Autodesk Fusion 360 part; units mm, degrees
(part 9 of 9)
  line L288 (-3.2885, -31.7147) -> (2.6698, -31.7147) construction
  line L289 (2.6698, -31.7147) -> (2.6698, -21.1314) construction
  line L290 (2.6698, -21.1314) -> (-3.2885, -21.1314) construction
  line L291 (-3.2885, -21.1314) -> (-3.2885, -31.7147) construction
  line L292 (13.3802, -31.7147) -> (19.3488, -31.7147) construction
  line L293 (19.3488, -31.7147) -> (19.3488, -21.1314) construction
  line L294 (19.3488, -21.1314) -> (13.3802, -21.1314) construction
  line L295 (13.3802, -21.1314) -> (13.3802, -31.7147) construction
  line L296 (30.049, -31.7147) -> (36.3121, -31.7147) construction
  line L297 (36.3121, -31.7147) -> (36.3121, -21.1314) construction
  line L298 (36.3121, -21.1314) -> (30.049, -21.1314) construction
  line L299 (30.049, -21.1314) -> (30.049, -31.7147) construction
  line L300 (46.7177, -31.7147) -> (53.3943, -31.7147) construction
  line L301 (53.3943, -31.7147) -> (53.3943, -21.1314) construction
  line L302 (53.3943, -21.1314) -> (46.7177, -21.1314) construction
  line L303 (46.7177, -21.1314) -> (46.7177, -31.7147) construction
  line L304 (63.3865, -31.7147) -> (69.0399, -31.7147) construction
  line L305 (69.0399, -31.7147) -> (69.0399, -21.1314) construction
  line L306 (69.0399, -21.1314) -> (63.3865, -21.1314) construction
  line L307 (63.3865, -21.1314) -> (63.3865, -31.7147) construction
  line L308 (80.0552, -31.7147) -> (81.0577, -31.7147) construction
  line L309 (81.0577, -31.7147) -> (81.0577, -21.1314) construction
  line L310 (81.0577, -21.1314) -> (80.0552, -21.1314) construction
  line L311 (80.0552, -21.1314) -> (80.0552, -31.7147) construction
  line L312 (-86.6323, -50.2147) -> (-80.643, -50.2147) construction
  line L313 (-80.643, -50.2147) -> (-80.643, -39.6314) construction
  line L314 (-80.643, -39.6314) -> (-86.6323, -39.6314) construction
  line L315 (-86.6323, -39.6314) -> (-86.6323, -50.2147) construction
  line L316 (-69.9635, -50.2147) -> (-60.2225, -50.2147) construction
  line L317 (-60.2225, -50.2147) -> (-60.2225, -39.6314) construction
  line L318 (-60.2225, -39.6314) -> (-69.9635, -39.6314) construction
  line L319 (-69.9635, -39.6314) -> (-69.9635, -50.2147) construction
  line L320 (-53.2948, -50.2147) -> (-47.6414, -50.2147) construction
  line L321 (-47.6414, -50.2147) -> (-47.6414, -39.6314) construction
  line L322 (-47.6414, -39.6314) -> (-53.2948, -39.6314) construction
  line L323 (-53.2948, -39.6314) -> (-53.2948, -50.2147) construction
  line L324 (-36.626, -50.2147) -> (-35.6235, -50.2147) construction
  line L325 (-35.6235, -50.2147) -> (-35.6235, -39.6314) construction
  line L326 (-35.6235, -39.6314) -> (-36.626, -39.6314) construction
  line L327 (-36.626, -39.6314) -> (-36.626, -50.2147) construction
  line L328 (-19.9573, -50.2147) -> (-13.9887, -50.2147) construction
  line L329 (-13.9887, -50.2147) -> (-13.9887, -39.6314) construction
  line L330 (-13.9887, -39.6314) -> (-19.9573, -39.6314) construction
  line L331 (-19.9573, -39.6314) -> (-19.9573, -50.2147) construction
  line L332 (-3.2885, -50.2147) -> (2.7421, -50.2147) construction
  line L333 (2.7421, -50.2147) -> (2.7421, -39.6314) construction
  line L334 (2.7421, -39.6314) -> (-3.2885, -39.6314) construction
  line L335 (-3.2885, -39.6314) -> (-3.2885, -50.2147) construction
  line L336 (13.3802, -50.2147) -> (14.3827, -50.2147) construction
  line L337 (14.3827, -50.2147) -> (14.3827, -39.6314) construction
  line L338 (14.3827, -39.6314) -> (13.3802, -39.6314) construction
  line L339 (13.3802, -39.6314) -> (13.3802, -50.2147) construction
  line L340 (30.049, -50.2147) -> (35.7024, -50.2147) construction
  line L341 (35.7024, -50.2147) -> (35.7024, -39.6314) construction
  line L342 (35.7024, -39.6314) -> (30.049, -39.6314) construction
  line L343 (30.049, -39.6314) -> (30.049, -50.2147) construction
  line L344 (46.7177, -50.2147) -> (52.4383, -50.2147) construction
  line L345 (52.4383, -50.2147) -> (52.4383, -39.6314) construction
  line L346 (52.4383, -39.6314) -> (46.7177, -39.6314) construction
  line L347 (46.7177, -39.6314) -> (46.7177, -50.2147) construction
  line L348 (63.3865, -50.2147) -> (69.0399, -50.2147) construction
  line L349 (69.0399, -50.2147) -> (69.0399, -39.6314) construction
  line L350 (69.0399, -39.6314) -> (63.3865, -39.6314) construction
  line L351 (63.3865, -39.6314) -> (63.3865, -50.2147) construction
  line L352 (80.0552, -50.2147) -> (86.0238, -50.2147) construction
  line L353 (86.0238, -50.2147) -> (86.0238, -39.6314) construction
  line L354 (86.0238, -39.6314) -> (80.0552, -39.6314) construction
  line L355 (80.0552, -39.6314) -> (80.0552, -50.2147) construction
  line L356 (-86.6323, -68.7148) -> (-80.9789, -68.7148) construction
  line L357 (-80.9789, -68.7148) -> (-80.9789, -58.1314) construction
  line L358 (-80.9789, -58.1314) -> (-86.6323, -58.1314) construction
  line L359 (-86.6323, -58.1314) -> (-86.6323, -68.7148) construction
  line L360 (-69.9635, -68.7148) -> (-65.23, -68.7148) construction
  line L361 (-65.23, -68.7148) -> (-65.23, -58.1314) construction
  line L362 (-65.23, -58.1314) -> (-69.9635, -58.1314) construction
  line L363 (-69.9635, -58.1314) -> (-69.9635, -68.7148) construction
  line L364 (-53.2948, -68.7148) -> (-48.184, -68.7148) construction
  line L365 (-48.184, -68.7148) -> (-48.184, -58.1314) construction
  line L366 (-48.184, -58.1314) -> (-53.2948, -58.1314) construction
  line L367 (-53.2948, -58.1314) -> (-53.2948, -68.7148) construction
  line L368 (-36.626, -68.7148) -> (-29.6962, -68.7148) construction
  line L369 (-29.6962, -68.7148) -> (-29.6962, -58.1314) construction
  line L370 (-29.6962, -58.1314) -> (-36.626, -58.1314) construction
  line L371 (-36.626, -58.1314) -> (-36.626, -68.7148) construction
  line L372 (-19.9573, -68.7148) -> (-18.9548, -68.7148) construction
  line L373 (-18.9548, -68.7148) -> (-18.9548, -58.1314) construction
  line L374 (-18.9548, -58.1314) -> (-19.9573, -58.1314) construction
  line L375 (-19.9573, -58.1314) -> (-19.9573, -68.7148) construction
  line L376 (-3.2885, -68.7148) -> (2.3649, -68.7148) construction
  line L377 (2.3649, -68.7148) -> (2.3649, -58.1314) construction
  line L378 (2.3649, -58.1314) -> (-3.2885, -58.1314) construction
  line L379 (-3.2885, -58.1314) -> (-3.2885, -68.7148) construction
  line L380 (13.3802, -68.7148) -> (20.0568, -68.7148) construction
  line L381 (20.0568, -68.7148) -> (20.0568, -58.1314) construction
  line L382 (20.0568, -58.1314) -> (13.3802, -58.1314) construction
  line L383 (13.3802, -58.1314) -> (13.3802, -68.7148) construction
  line L384 (30.049, -68.7148) -> (37.139, -68.7148) construction
  line L385 (37.139, -68.7148) -> (37.139, -58.1314) construction
  line L386 (37.139, -58.1314) -> (30.049, -58.1314) construction
  line L387 (30.049, -58.1314) -> (30.049, -68.7148) construction
  line L388 (46.7177, -68.7148) -> (53.415, -68.7148) construction
  line L389 (53.415, -68.7148) -> (53.415, -58.1314) construction
  line L390 (53.415, -58.1314) -> (46.7177, -58.1314) construction
  line L391 (46.7177, -58.1314) -> (46.7177, -68.7148) construction
  line L392 (63.3865, -68.7148) -> (69.3292, -68.7148) construction
  line L393 (69.3292, -68.7148) -> (69.3292, -58.1314) construction
  line L394 (69.3292, -58.1314) -> (63.3865, -58.1314) construction
  line L395 (63.3865, -58.1314) -> (63.3865, -68.7148) construction
  line L396 (80.0552, -68.7148) -> (86.06, -68.7148) construction
  line L397 (86.06, -68.7148) -> (86.06, -58.1314) construction
  line L398 (86.06, -58.1314) -> (80.0552, -58.1314) construction
  line L399 (80.0552, -58.1314) -> (80.0552, -68.7148) construction
  line L400 (-86.6323, -87.2148) -> (-80.6017, -87.2148) construction
  line L401 (-80.6017, -87.2148) -> (-80.6017, -76.6314) construction
  line L402 (-80.6017, -76.6314) -> (-86.6323, -76.6314) construction
  line L403 (-86.6323, -76.6314) -> (-86.6323, -87.2148) construction
  line L404 (-69.9635, -87.2148) -> (-64.3101, -87.2148) construction
  line L405 (-64.3101, -87.2148) -> (-64.3101, -76.6314) construction
  line L406 (-64.3101, -76.6314) -> (-69.9635, -76.6314) construction
  line L407 (-69.9635, -76.6314) -> (-69.9635, -87.2148) construction
  line L408 (-53.2948, -87.2148) -> (-46.5975, -87.2148) construction
  line L409 (-46.5975, -87.2148) -> (-46.5975, -76.6314) construction
  line L410 (-46.5975, -76.6314) -> (-53.2948, -76.6314) construction
  line L411 (-53.2948, -76.6314) -> (-53.2948, -87.2148) construction
  line L412 (-36.626, -87.2148) -> (-30.6833, -87.2148) construction
  line L413 (-30.6833, -87.2148) -> (-30.6833, -76.6314) construction
  line L414 (-30.6833, -76.6314) -> (-36.626, -76.6314) construction
  line L415 (-36.626, -76.6314) -> (-36.626, -87.2148) construction
  line L416 (-19.9573, -87.2148) -> (-13.9267, -87.2148) construction
  line L417 (-13.9267, -87.2148) -> (-13.9267, -76.6314) construction
  line L418 (-13.9267, -76.6314) -> (-19.9573, -76.6314) construction
  line L419 (-19.9573, -76.6314) -> (-19.9573, -87.2148) construction
  line L420 (-3.2885, -87.2148) -> (-2.286, -87.2148) construction
  line L421 (-2.286, -87.2148) -> (-2.286, -76.6314) construction
  line L422 (-2.286, -76.6314) -> (-3.2885, -76.6314) construction
  line L423 (-3.2885, -76.6314) -> (-3.2885, -87.2148) construction
  line L424 (13.3802, -87.2148) -> (19.3385, -87.2148) construction
  line L425 (19.3385, -87.2148) -> (19.3385, -76.6314) construction
  line L426 (19.3385, -76.6314) -> (13.3802, -76.6314) construction
  line L427 (13.3802, -76.6314) -> (13.3802, -87.2148) construction
  line L428 (30.049, -87.2148) -> (35.9917, -87.2148) construction
  line L429 (35.9917, -87.2148) -> (35.9917, -76.6314) construction
  line L430 (35.9917, -76.6314) -> (30.049, -76.6314) construction
  line L431 (30.049, -76.6314) -> (30.049, -87.2148) construction
  line L432 (46.7177, -87.2148) -> (53.3943, -87.2148) construction
  line L433 (53.3943, -87.2148) -> (53.3943, -76.6314) construction
  line L434 (53.3943, -76.6314) -> (46.7177, -76.6314) construction
  line L435 (46.7177, -76.6314) -> (46.7177, -87.2148) construction
  line L436 (63.3865, -87.2148) -> (70.3318, -87.2148) construction
  line L437 (70.3318, -87.2148) -> (70.3318, -76.6314) construction
  line L438 (70.3318, -76.6314) -> (63.3865, -76.6314) construction
  line L439 (63.3865, -76.6314) -> (63.3865, -87.2148) construction
  line L440 (80.0552, -87.2148) -> (85.7086, -87.2148) construction
  line L441 (85.7086, -87.2148) -> (85.7086, -76.6314) construction
  line L442 (85.7086, -76.6314) -> (80.0552, -76.6314) construction
  line L443 (80.0552, -76.6314) -> (80.0552, -87.2148) construction
sketch "Sketch6" plane through (0, 0, 7) normal (0, 0, 1) x (-1, 0, 0)
  line L0 (57.9, 38.615) -> (42.9, 38.615)
  line L1 (42.9, 38.615) -> (42.9, 53.615)
  line L2 (42.9, 53.615) -> (57.9, 53.615)
  line L3 (57.9, 53.615) -> (57.9, 38.615)
  line L4 (-9.3, 20.17) -> (-24.3, 20.17)
  line L5 (-24.3, 20.17) -> (-24.3, 35.17)
  line L6 (-24.3, 35.17) -> (-9.3, 35.17)
  line L7 (-9.3, 35.17) -> (-9.3, 20.17)
  line L8 (-26.1, 20.17) -> (-41.1, 20.17)
  line L9 (-41.1, 20.17) -> (-41.1, 35.17)
  line L10 (-41.1, 35.17) -> (-26.1, 35.17)
  line L11 (-26.1, 35.17) -> (-26.1, 20.17)
  line L12 (-42.9, 20.17) -> (-57.9, 20.17)
  line L13 (-57.9, 20.17) -> (-57.9, 35.17)
  line L14 (-57.9, 35.17) -> (-42.9, 35.17)
  line L15 (-42.9, 35.17) -> (-42.9, 20.17)
  line L16 (-59.7, 1.725) -> (-74.7, 1.725)
  line L17 (-74.7, 1.725) -> (-74.7, 16.725)
  line L18 (-74.7, 16.725) -> (-59.7, 16.725)
  line L19 (-59.7, 16.725) -> (-59.7, 1.725)
  line L20 (7.5, 1.725) -> (-7.5, 1.725)
  line L21 (-7.5, 1.725) -> (-7.5, 16.725)
  line L22 (-7.5, 16.725) -> (7.5, 16.725)
  line L23 (7.5, 16.725) -> (7.5, 1.725)
  line L24 (-59.7, 20.17) -> (-74.7, 20.17)
  line L25 (-74.7, 20.17) -> (-74.7, 35.17)
  line L26 (-74.7, 35.17) -> (-59.7, 35.17)
  line L27 (-59.7, 35.17) -> (-59.7, 20.17)
  line L28 (57.9, 1.725) -> (42.9, 1.725)
  line L29 (42.9, 1.725) -> (42.9, 16.725)
  line L30 (42.9, 16.725) -> (57.9, 16.725)
  line L31 (57.9, 16.725) -> (57.9, 1.725)
  line L32 (41.1, 38.615) -> (26.1, 38.615)
  line L33 (26.1, 38.615) -> (26.1, 53.615)
  line L34 (26.1, 53.615) -> (41.1, 53.615)
  line L35 (41.1, 53.615) -> (41.1, 38.615)
  line L36 (41.1, 1.725) -> (26.1, 1.725)
  line L37 (26.1, 1.725) -> (26.1, 16.725)
  line L38 (26.1, 16.725) -> (41.1, 16.725)
  line L39 (41.1, 16.725) -> (41.1, 1.725)
  line L40 (-76.5, 1.725) -> (-91.5, 1.725)
  line L41 (-91.5, 1.725) -> (-91.5, 16.725)
  line L42 (-91.5, 16.725) -> (-76.5, 16.725)
  line L43 (-76.5, 16.725) -> (-76.5, 1.725)
  line L44 (24.3, 1.725) -> (9.3, 1.725)
  line L45 (9.3, 1.725) -> (9.3, 16.725)
  line L46 (9.3, 16.725) -> (24.3, 16.725)
  line L47 (24.3, 16.725) -> (24.3, 1.725)
  line L48 (-76.5, 20.17) -> (-91.5, 20.17)
  line L49 (-91.5, 20.17) -> (-91.5, 35.17)
  line L50 (-91.5, 35.17) -> (-76.5, 35.17)
  line L51 (-76.5, 35.17) -> (-76.5, 20.17)
  line L52 (-59.7, -53.61) -> (-74.7, -53.61)
  line L53 (-74.7, -53.61) -> (-74.7, -38.61)
  line L54 (-74.7, -38.61) -> (-59.7, -38.61)
  line L55 (-59.7, -38.61) -> (-59.7, -53.61)
  line L56 (-76.5, -53.61) -> (-91.5, -53.61)
  line L57 (-91.5, -53.61) -> (-91.5, -38.61)
  line L58 (-91.5, -38.61) -> (-76.5, -38.61)
  line L59 (-76.5, -38.61) -> (-76.5, -53.61)
  line L60 (-42.9, -53.61) -> (-57.9, -53.61)
  line L61 (-57.9, -53.61) -> (-57.9, -38.61)
  line L62 (-57.9, -38.61) -> (-42.9, -38.61)
  line L63 (-42.9, -38.61) -> (-42.9, -53.61)
  line L64 (41.1, -16.72) -> (26.1, -16.72)
  line L65 (26.1, -16.72) -> (26.1, -1.72)
  line L66 (26.1, -1.72) -> (41.1, -1.72)
  line L67 (41.1, -1.72) -> (41.1, -16.72)
  line L68 (-26.1, -53.61) -> (-41.1, -53.61)
  line L69 (-41.1, -53.61) -> (-41.1, -38.61)
  line L70 (-41.1, -38.61) -> (-26.1, -38.61)
  line L71 (-26.1, -38.61) -> (-26.1, -53.61)
  line L72 (-9.3, -35.165) -> (-24.3, -35.165)
  line L73 (-24.3, -35.165) -> (-24.3, -20.165)
  line L74 (-24.3, -20.165) -> (-9.3, -20.165)
  line L75 (-9.3, -20.165) -> (-9.3, -35.165)
  line L76 (91.5, -35.165) -> (76.5, -35.165)
  line L77 (76.5, -35.165) -> (76.5, -20.165)
  line L78 (76.5, -20.165) -> (91.5, -20.165)
  line L79 (91.5, -20.165) -> (91.5, -35.165)
  line L80 (91.5, 38.615) -> (76.5, 38.615)
  line L81 (76.5, 38.615) -> (76.5, 53.615)
  line L82 (76.5, 53.615) -> (91.5, 53.615)
  line L83 (91.5, 53.615) -> (91.5, 38.615)
  line L84 (-9.3, -16.72) -> (-24.3, -16.72)
  line L85 (-24.3, -16.72) -> (-24.3, -1.72)
  line L86 (-24.3, -1.72) -> (-9.3, -1.72)
  line L87 (-9.3, -1.72) -> (-9.3, -16.72)
  line L88 (74.7, 38.615) -> (59.7, 38.615)
  line L89 (59.7, 38.615) -> (59.7, 53.615)
  line L90 (59.7, 53.615) -> (74.7, 53.615)
  line L91 (74.7, 53.615) -> (74.7, 38.615)
  line L92 (-9.3, 1.725) -> (-24.3, 1.725)
  line L93 (-24.3, 1.725) -> (-24.3, 16.725)
  line L94 (-24.3, 16.725) -> (-9.3, 16.725)
  line L95 (-9.3, 16.725) -> (-9.3, 1.725)
  line L96 (-42.9, -16.72) -> (-57.9, -16.72)
  line L97 (-57.9, -16.72) -> (-57.9, -1.72)
  line L98 (-57.9, -1.72) -> (-42.9, -1.72)
  line L99 (-42.9, -1.72) -> (-42.9, -16.72)
  line L100 (7.5, -16.72) -> (-7.5, -16.72)
  line L101 (-7.5, -16.72) -> (-7.5, -1.72)
  line L102 (-7.5, -1.72) -> (7.5, -1.72)
  line L103 (7.5, -1.72) -> (7.5, -16.72)
  line L104 (-26.1, -16.72) -> (-41.1, -16.72)
  line L105 (-41.1, -16.72) -> (-41.1, -1.72)
  line L106 (-41.1, -1.72) -> (-26.1, -1.72)
  line L107 (-26.1, -1.72) -> (-26.1, -16.72)
  line L108 (-59.7, -16.72) -> (-74.7, -16.72)
  line L109 (-74.7, -16.72) -> (-74.7, -1.72)
  line L110 (-74.7, -1.72) -> (-59.7, -1.72)
  line L111 (-59.7, -1.72) -> (-59.7, -16.72)
  line L112 (91.5, -16.72) -> (76.5, -16.72)
  line L113 (76.5, -16.72) -> (76.5, -1.72)
  line L114 (76.5, -1.72) -> (91.5, -1.72)
  line L115 (91.5, -1.72) -> (91.5, -16.72)
  line L116 (-76.5, -16.72) -> (-91.5, -16.72)
  line L117 (-91.5, -16.72) -> (-91.5, -1.72)
  line L118 (-91.5, -1.72) -> (-76.5, -1.72)
  line L119 (-76.5, -1.72) -> (-76.5, -16.72)
  line L120 (74.7, -16.72) -> (59.7, -16.72)
  line L121 (59.7, -16.72) -> (59.7, -1.72)
  line L122 (59.7, -1.72) -> (74.7, -1.72)
  line L123 (74.7, -1.72) -> (74.7, -16.72)
  line L124 (91.5, 20.17) -> (76.5, 20.17)
  line L125 (76.5, 20.17) -> (76.5, 35.17)
  line L126 (76.5, 35.17) -> (91.5, 35.17)
  line L127 (91.5, 35.17) -> (91.5, 20.17)
  line L128 (-42.9, -35.165) -> (-57.9, -35.165)
  line L129 (-57.9, -35.165) -> (-57.9, -20.165)
  line L130 (-57.9, -20.165) -> (-42.9, -20.165)
  line L131 (-42.9, -20.165) -> (-42.9, -35.165)
  line L132 (-59.7, -35.165) -> (-74.7, -35.165)
  line L133 (-74.7, -35.165) -> (-74.7, -20.165)
  line L134 (-74.7, -20.165) -> (-59.7, -20.165)
  line L135 (-59.7, -20.165) -> (-59.7, -35.165)
  line L136 (91.5, 1.725) -> (76.5, 1.725)
  line L137 (76.5, 1.725) -> (76.5, 16.725)
  line L138 (76.5, 16.725) -> (91.5, 16.725)
  line L139 (91.5, 16.725) -> (91.5, 1.725)
  line L140 (24.3, -35.165) -> (9.3, -35.165)
  line L141 (9.3, -35.165) -> (9.3, -20.165)
  line L142 (9.3, -20.165) -> (24.3, -20.165)
  line L143 (24.3, -20.165) -> (24.3, -35.165)
  line L144 (7.5, -35.165) -> (-7.5, -35.165)
  line L145 (-7.5, -35.165) -> (-7.5, -20.165)
  line L146 (-7.5, -20.165) -> (7.5, -20.165)
  line L147 (7.5, -20.165) -> (7.5, -35.165)
  line L148 (57.9, -16.72) -> (42.9, -16.72)
  line L149 (42.9, -16.72) -> (42.9, -1.72)
  line L150 (42.9, -1.72) -> (57.9, -1.72)
  line L151 (57.9, -1.72) -> (57.9, -16.72)
  line L152 (-26.1, 1.725) -> (-41.1, 1.725)
  line L153 (-41.1, 1.725) -> (-41.1, 16.725)
  line L154 (-41.1, 16.725) -> (-26.1, 16.725)
  line L155 (-26.1, 16.725) -> (-26.1, 1.725)
  line L156 (41.1, -35.165) -> (26.1, -35.165)
  line L157 (26.1, -35.165) -> (26.1, -20.165)
  line L158 (26.1, -20.165) -> (41.1, -20.165)
  line L159 (41.1, -20.165) -> (41.1, -35.165)
  line L160 (-9.3, -53.61) -> (-24.3, -53.61)
  line L161 (-24.3, -53.61) -> (-24.3, -38.61)
  line L162 (-24.3, -38.61) -> (-9.3, -38.61)
  line L163 (-9.3, -38.61) -> (-9.3, -53.61)
  line L164 (-26.1, -72.055) -> (-41.1, -72.055)
  line L165 (-41.1, -72.055) -> (-41.1, -57.055)
  line L166 (-41.1, -57.055) -> (-26.1, -57.055)
  line L167 (-26.1, -57.055) -> (-26.1, -72.055)
  line L168 (-26.1, -90.5) -> (-41.1, -90.5)
  line L169 (-41.1, -90.5) -> (-41.1, -75.5)
  line L170 (-41.1, -75.5) -> (-26.1, -75.5)
  line L171 (-26.1, -75.5) -> (-26.1, -90.5)
  line L172 (-9.3, -90.5) -> (-24.3, -90.5)
  line L173 (-24.3, -90.5) -> (-24.3, -75.5)
  line L174 (-24.3, -75.5) -> (-9.3, -75.5)
  line L175 (-9.3, -75.5) -> (-9.3, -90.5)
  line L176 (7.5, -53.61) -> (-7.5, -53.61)
  line L177 (-7.5, -53.61) -> (-7.5, -38.61)
  line L178 (-7.5, -38.61) -> (7.5, -38.61)
  line L179 (7.5, -38.61) -> (7.5, -53.61)
  line L180 (7.5, -90.5) -> (-7.5, -90.5)
  line L181 (-7.5, -90.5) -> (-7.5, -75.5)
  line L182 (-7.5, -75.5) -> (7.5, -75.5)
  line L183 (7.5, -75.5) -> (7.5, -90.5)
  line L184 (24.3, -90.5) -> (9.3, -90.5)
  line L185 (9.3, -90.5) -> (9.3, -75.5)
  line L186 (9.3, -75.5) -> (24.3, -75.5)
  line L187 (24.3, -75.5) -> (24.3, -90.5)
  line L188 (57.9, -35.165) -> (42.9, -35.165)
  line L189 (42.9, -35.165) -> (42.9, -20.165)
  line L190 (42.9, -20.165) -> (57.9, -20.165)
  line L191 (57.9, -20.165) -> (57.9, -35.165)
  line L192 (-42.9, 1.725) -> (-57.9, 1.725)
  line L193 (-57.9, 1.725) -> (-57.9, 16.725)
  line L194 (-57.9, 16.725) -> (-42.9, 16.725)
  line L195 (-42.9, 16.725) -> (-42.9, 1.725)
  line L196 (91.5, -72.055) -> (76.5, -72.055)
  line L197 (76.5, -72.055) -> (76.5, -57.055)
  line L198 (76.5, -57.055) -> (91.5, -57.055)
  line L199 (91.5, -57.055) -> (91.5, -72.055)
  line L200 (-42.9, -72.055) -> (-57.9, -72.055)
  line L201 (-57.9, -72.055) -> (-57.9, -57.055)
  line L202 (-57.9, -57.055) -> (-42.9, -57.055)
  line L203 (-42.9, -57.055) -> (-42.9, -72.055)
  line L204 (74.7, 1.725) -> (59.7, 1.725)
  line L205 (59.7, 1.725) -> (59.7, 16.725)
  line L206 (59.7, 16.725) -> (74.7, 16.725)
  line L207 (74.7, 16.725) -> (74.7, 1.725)
  line L208 (74.7, -53.61) -> (59.7, -53.61)
  line L209 (59.7, -53.61) -> (59.7, -38.61)
  line L210 (59.7, -38.61) -> (74.7, -38.61)
  line L211 (74.7, -38.61) -> (74.7, -53.61)
  line L212 (91.5, -53.61) -> (76.5, -53.61)
  line L213 (76.5, -53.61) -> (76.5, -38.61)
  line L214 (76.5, -38.61) -> (91.5, -38.61)
  line L215 (91.5, -38.61) -> (91.5, -53.61)
  line L216 (-76.5, -72.055) -> (-91.5, -72.055)
  line L217 (-91.5, -72.055) -> (-91.5, -57.055)
  line L218 (-91.5, -57.055) -> (-76.5, -57.055)
  line L219 (-76.5, -57.055) -> (-76.5, -72.055)
  line L220 (74.7, -35.165) -> (59.7, -35.165)
  line L221 (59.7, -35.165) -> (59.7, -20.165)
  line L222 (59.7, -20.165) -> (74.7, -20.165)
  line L223 (74.7, -20.165) -> (74.7, -35.165)
  line L224 (-26.1, -35.165) -> (-41.1, -35.165)
  line L225 (-41.1, -35.165) -> (-41.1, -20.165)
  line L226 (-41.1, -20.165) -> (-26.1, -20.165)
  line L227 (-26.1, -20.165) -> (-26.1, -35.165)
  line L228 (76.5, -75.5) -> (91.5, -75.5)
  line L229 (91.5, -75.5) -> (91.5, -90.5)
  line L230 (91.5, -90.5) -> (76.5, -90.5)
  line L231 (76.5, -90.5) -> (76.5, -75.5)
  circle A0 centre (110, -110) radius 1.6
  circle A1 centre (-110, 110) radius 1.6
  line L232 (57.9, -53.61) -> (42.9, -53.61)
  line L233 (42.9, -53.61) -> (42.9, -38.61)
  line L234 (42.9, -38.61) -> (57.9, -38.61)
  line L235 (57.9, -38.61) -> (57.9, -53.61)
  circle A2 centre (110, 110) radius 1.6
  line L236 (74.7, -90.5) -> (59.7, -90.5)
  line L237 (59.7, -90.5) -> (59.7, -75.5)
  line L238 (59.7, -75.5) -> (74.7, -75.5)
  line L239 (74.7, -75.5) -> (74.7, -90.5)
  circle A3 centre (-110, -110) radius 1.6
  line L240 (41.1, -90.5) -> (26.1, -90.5)
  line L241 (26.1, -90.5) -> (26.1, -75.5)
  line L242 (26.1, -75.5) -> (41.1, -75.5)
  line L243 (41.1, -75.5) -> (41.1, -90.5)
  line L244 (41.1, -53.61) -> (26.1, -53.61)
  line L245 (26.1, -53.61) -> (26.1, -38.61)
  line L246 (26.1, -38.61) -> (41.1, -38.61)
  line L247 (41.1, -38.61) -> (41.1, -53.61)
  line L248 (-76.5, -90.5) -> (-91.5, -90.5)
  line L249 (-91.5, -90.5) -> (-91.5, -75.5)
  line L250 (-91.5, -75.5) -> (-76.5, -75.5)
  line L251 (-76.5, -75.5) -> (-76.5, -90.5)
  line L252 (-59.7, -90.5) -> (-74.7, -90.5)
  line L253 (-74.7, -90.5) -> (-74.7, -75.5)
  line L254 (-74.7, -75.5) -> (-59.7, -75.5)
  line L255 (-59.7, -75.5) -> (-59.7, -90.5)
  line L256 (24.3, -16.72) -> (9.3, -16.72)
  line L257 (9.3, -16.72) -> (9.3, -1.72)
  line L258 (9.3, -1.72) -> (24.3, -1.72)
  line L259 (24.3, -1.72) -> (24.3, -16.72)
  line L260 (-59.7, -72.055) -> (-74.7, -72.055)
  line L261 (-74.7, -72.055) -> (-74.7, -57.055)
  line L262 (-74.7, -57.055) -> (-59.7, -57.055)
  line L263 (-59.7, -57.055) -> (-59.7, -72.055)
  line L264 (-76.5, -35.165) -> (-91.5, -35.165)
  line L265 (-91.5, -35.165) -> (-91.5, -20.165)
  line L266 (-91.5, -20.165) -> (-76.5, -20.165)
  line L267 (-76.5, -20.165) -> (-76.5, -35.165)
  line L268 (74.7, -72.055) -> (59.7, -72.055)
  line L269 (59.7, -72.055) -> (59.7, -57.055)
  line L270 (59.7, -57.055) -> (74.7, -57.055)
  line L271 (74.7, -57.055) -> (74.7, -72.055)
  line L272 (57.9, -90.5) -> (42.9, -90.5)
  line L273 (42.9, -90.5) -> (42.9, -75.5)
  line L274 (42.9, -75.5) -> (57.9, -75.5)
  line L275 (57.9, -75.5) -> (57.9, -90.5)
  line L276 (24.3, -53.61) -> (9.3, -53.61)
  line L277 (9.3, -53.61) -> (9.3, -38.61)
  line L278 (9.3, -38.61) -> (24.3, -38.61)
  line L279 (24.3, -38.61) -> (24.3, -53.61)
  line L280 (-42.9, -90.5) -> (-57.9, -90.5)
  line L281 (-57.9, -90.5) -> (-57.9, -75.5)
  line L282 (-57.9, -75.5) -> (-42.9, -75.5)
  line L283 (-42.9, -75.5) -> (-42.9, -90.5)
  line L284 (57.9, 75.505) -> (42.9, 75.505)
  line L285 (42.9, 75.505) -> (42.9, 90.505)
  line L286 (42.9, 90.505) -> (57.9, 90.505)
  line L287 (57.9, 90.505) -> (57.9, 75.505)
  line L288 (7.5, 75.505) -> (-7.5, 75.505)
  line L289 (-7.5, 75.505) -> (-7.5, 90.505)
  line L290 (-7.5, 90.505) -> (7.5, 90.505)
  line L291 (7.5, 90.505) -> (7.5, 75.505)
  line L292 (-26.1, 75.505) -> (-41.1, 75.505)
  line L293 (-41.1, 75.505) -> (-41.1, 90.505)
  line L294 (-41.1, 90.505) -> (-26.1, 90.505)
  line L295 (-26.1, 90.505) -> (-26.1, 75.505)
  line L296 (24.3, 75.505) -> (9.3, 75.505)
  line L297 (9.3, 75.505) -> (9.3, 90.505)
  line L298 (9.3, 90.505) -> (24.3, 90.505)
  line L299 (24.3, 90.505) -> (24.3, 75.505)
  line L300 (74.7, 75.505) -> (59.7, 75.505)
  line L301 (59.7, 75.505) -> (59.7, 90.505)
  line L302 (59.7, 90.505) -> (74.7, 90.505)
  line L303 (74.7, 90.505) -> (74.7, 75.505)
  line L304 (41.1, 75.505) -> (26.1, 75.505)
  line L305 (26.1, 75.505) -> (26.1, 90.505)
  line L306 (26.1, 90.505) -> (41.1, 90.505)
  line L307 (41.1, 90.505) -> (41.1, 75.505)
  line L308 (91.5, 75.505) -> (76.5, 75.505)
  line L309 (76.5, 75.505) -> (76.5, 90.505)
  line L310 (76.5, 90.505) -> (91.5, 90.505)
  line L311 (91.5, 90.505) -> (91.5, 75.505)
  line L312 (-9.3, 75.505) -> (-24.3, 75.505)
  line L313 (-24.3, 75.505) -> (-24.3, 90.505)
  line L314 (-24.3, 90.505) -> (-9.3, 90.505)
  line L315 (-9.3, 90.505) -> (-9.3, 75.505)
  line L316 (-76.5, 57.06) -> (-91.5, 57.06)
  line L317 (-91.5, 57.06) -> (-91.5, 72.06)
  line L318 (-91.5, 72.06) -> (-76.5, 72.06)
  line L319 (-76.5, 72.06) -> (-76.5, 57.06)
  line L320 (-42.9, 57.06) -> (-57.9, 57.06)
  line L321 (-57.9, 57.06) -> (-57.9, 72.06)
  line L322 (-57.9, 72.06) -> (-42.9, 72.06)
  line L323 (-42.9, 72.06) -> (-42.9, 57.06)
  line L324 (-59.7, 57.06) -> (-74.7, 57.06)
  line L325 (-74.7, 57.06) -> (-74.7, 72.06)
  line L326 (-74.7, 72.06) -> (-59.7, 72.06)
  line L327 (-59.7, 72.06) -> (-59.7, 57.06)
  line L328 (24.175, 99.3) -> (9.175, 99.3)
  line L329 (9.175, 99.3) -> (9.175, 114.3)
  line L330 (9.175, 114.3) -> (24.175, 114.3)
  line L331 (24.175, 114.3) -> (24.175, 99.3)
  line L332 (7.5, -72.055) -> (-7.5, -72.055)
  line L333 (-7.5, -72.055) -> (-7.5, -57.055)
  line L334 (-7.5, -57.055) -> (7.5, -57.055)
  line L335 (7.5, -57.055) -> (7.5, -72.055)
  line L336 (-42.475, 99.3) -> (-57.475, 99.3)
  line L337 (-57.475, 99.3) -> (-57.475, 114.3)
  line L338 (-57.475, 114.3) -> (-42.475, 114.3)
  line L339 (-42.475, 114.3) -> (-42.475, 99.3)
  line L340 (-9.3, 57.06) -> (-24.3, 57.06)
  line L341 (-24.3, 57.06) -> (-24.3, 72.06)
  line L342 (-24.3, 72.06) -> (-9.3, 72.06)
  line L343 (-9.3, 72.06) -> (-9.3, 57.06)
  line L344 (7.5, 38.615) -> (-7.5, 38.615)
  line L345 (-7.5, 38.615) -> (-7.5, 53.615)
  line L346 (-7.5, 53.615) -> (7.5, 53.615)
  line L347 (7.5, 53.615) -> (7.5, 38.615)
  line L348 (-9.3, 38.615) -> (-24.3, 38.615)
  line L349 (-24.3, 38.615) -> (-24.3, 53.615)
  line L350 (-24.3, 53.615) -> (-9.3, 53.615)
  line L351 (-9.3, 53.615) -> (-9.3, 38.615)
  line L352 (24.3, 38.615) -> (9.3, 38.615)
  line L353 (9.3, 38.615) -> (9.3, 53.615)
  line L354 (9.3, 53.615) -> (24.3, 53.615)
  line L355 (24.3, 53.615) -> (24.3, 38.615)
  line L356 (-26.1, 38.615) -> (-41.1, 38.615)
  line L357 (-41.1, 38.615) -> (-41.1, 53.615)
  line L358 (-41.1, 53.615) -> (-26.1, 53.615)
  line L359 (-26.1, 53.615) -> (-26.1, 38.615)
  line L360 (91.5, 57.06) -> (76.5, 57.06)
  line L361 (76.5, 57.06) -> (76.5, 72.06)
  line L362 (76.5, 72.06) -> (91.5, 72.06)
  line L363 (91.5, 72.06) -> (91.5, 57.06)
  line L364 (24.3, 57.06) -> (9.3, 57.06)
  line L365 (9.3, 57.06) -> (9.3, 72.06)
  line L366 (9.3, 72.06) -> (24.3, 72.06)
  line L367 (24.3, 72.06) -> (24.3, 57.06)
  line L368 (-59.7, 38.615) -> (-74.7, 38.615)
  line L369 (-74.7, 38.615) -> (-74.7, 53.615)
  line L370 (-74.7, 53.615) -> (-59.7, 53.615)
  line L371 (-59.7, 53.615) -> (-59.7, 38.615)
  line L372 (41.1, 57.06) -> (26.1, 57.06)
  line L373 (26.1, 57.06) -> (26.1, 72.06)
  line L374 (26.1, 72.06) -> (41.1, 72.06)
  line L375 (41.1, 72.06) -> (41.1, 57.06)
  line L376 (57.9, 57.06) -> (42.9, 57.06)
  line L377 (42.9, 57.06) -> (42.9, 72.06)
  line L378 (42.9, 72.06) -> (57.9, 72.06)
  line L379 (57.9, 72.06) -> (57.9, 57.06)
  line L380 (-26.1, 57.06) -> (-41.1, 57.06)
  line L381 (-41.1, 57.06) -> (-41.1, 72.06)
  line L382 (-41.1, 72.06) -> (-26.1, 72.06)
  line L383 (-26.1, 72.06) -> (-26.1, 57.06)
  line L384 (7.5, 57.06) -> (-7.5, 57.06)
  line L385 (-7.5, 57.06) -> (-7.5, 72.06)
  line L386 (-7.5, 72.06) -> (7.5, 72.06)
  line L387 (7.5, 72.06) -> (7.5, 57.06)
  line L388 (7.5, 20.17) -> (-7.5, 20.17)
  line L389 (-7.5, 20.17) -> (-7.5, 35.17)
  line L390 (-7.5, 35.17) -> (7.5, 35.17)
  line L391 (7.5, 35.17) -> (7.5, 20.17)
  line L392 (-42.9, 38.615) -> (-57.9, 38.615)
  line L393 (-57.9, 38.615) -> (-57.9, 53.615)
  line L394 (-57.9, 53.615) -> (-42.9, 53.615)
  line L395 (-42.9, 53.615) -> (-42.9, 38.615)
  line L396 (24.3, 20.17) -> (9.3, 20.17)
  line L397 (9.3, 20.17) -> (9.3, 35.17)
  line L398 (9.3, 35.17) -> (24.3, 35.17)
  line L399 (24.3, 35.17) -> (24.3, 20.17)
  line L400 (57.9, 20.17) -> (42.9, 20.17)
  line L401 (42.9, 20.17) -> (42.9, 35.17)
  line L402 (42.9, 35.17) -> (57.9, 35.17)
  line L403 (57.9, 35.17) -> (57.9, 20.17)
  line L404 (74.7, 57.06) -> (59.7, 57.06)
  line L405 (59.7, 57.06) -> (59.7, 72.06)
  line L406 (59.7, 72.06) -> (74.7, 72.06)
  line L407 (74.7, 72.06) -> (74.7, 57.06)
  line L408 (-76.5, 38.615) -> (-91.5, 38.615)
  line L409 (-91.5, 38.615) -> (-91.5, 53.615)
  line L410 (-91.5, 53.615) -> (-76.5, 53.615)
  line L411 (-76.5, 53.615) -> (-76.5, 38.615)
  line L412 (-42.9, 75.505) -> (-57.9, 75.505)
  line L413 (-57.9, 75.505) -> (-57.9, 90.505)
  line L414 (-57.9, 90.505) -> (-42.9, 90.505)
  line L415 (-42.9, 90.505) -> (-42.9, 75.505)
  line L416 (41.1, -72.055) -> (26.1, -72.055)
  line L417 (26.1, -72.055) -> (26.1, -57.055)
  line L418 (26.1, -57.055) -> (41.1, -57.055)
  line L419 (41.1, -57.055) -> (41.1, -72.055)
  line L420 (74.7, 20.17) -> (59.7, 20.17)
  line L421 (59.7, 20.17) -> (59.7, 35.17)
  line L422 (59.7, 35.17) -> (74.7, 35.17)
  line L423 (74.7, 35.17) -> (74.7, 20.17)
  line L424 (41.1, 20.17) -> (26.1, 20.17)
  line L425 (26.1, 20.17) -> (26.1, 35.17)
  line L426 (26.1, 35.17) -> (41.1, 35.17)
  line L427 (41.1, 35.17) -> (41.1, 20.17)
  line L428 (-9.3, -72.055) -> (-24.3, -72.055)
  line L429 (-24.3, -72.055) -> (-24.3, -57.055)
  line L430 (-24.3, -57.055) -> (-9.3, -57.055)
  line L431 (-9.3, -57.055) -> (-9.3, -72.055)
  line L432 (-76.5, 75.505) -> (-91.5, 75.505)
  line L433 (-91.5, 75.505) -> (-91.5, 90.505)
  line L434 (-91.5, 90.505) -> (-76.5, 90.505)
  line L435 (-76.5, 90.505) -> (-76.5, 75.505)
  line L436 (24.3, -72.055) -> (9.3, -72.055)
  line L437 (9.3, -72.055) -> (9.3, -57.055)
  line L438 (9.3, -57.055) -> (24.3, -57.055)
  line L439 (24.3, -57.055) -> (24.3, -72.055)
  line L440 (57.9, -72.055) -> (42.9, -72.055)
  line L441 (42.9, -72.055) -> (42.9, -57.055)
  line L442 (42.9, -57.055) -> (57.9, -57.055)
  line L443 (57.9, -57.055) -> (57.9, -72.055)
  line L444 (-59.7, 75.505) -> (-74.7, 75.505)
  line L445 (-74.7, 75.505) -> (-74.7, 90.505)
  line L446 (-74.7, 90.505) -> (-59.7, 90.505)
  line L447 (-59.7, 90.505) -> (-59.7, 75.505)
  line L448 (-9.15, 99.3) -> (-24.15, 99.3)
  line L449 (-24.15, 99.3) -> (-24.15, 114.3)
  line L450 (-24.15, 114.3) -> (-9.15, 114.3)
  line L451 (-9.15, 114.3) -> (-9.15, 99.3)
  line L452 (42.5, 114.3) -> (57.5, 114.3)
  line L453 (57.5, 114.3) -> (57.5, 99.3)
  line L454 (57.5, 99.3) -> (42.5, 99.3)
  line L455 (42.5, 99.3) -> (42.5, 114.3)
  line L456 (-117.5, 117.5) -> (-117.5, -117.5)
  line L457 (-117.5, -117.5) -> (117.5, -117.5)
  line L458 (117.5, -117.5) -> (117.5, 117.5)
  line L459 (117.5, 117.5) -> (-117.5, 117.5)
  line L460 (117.5, -117.5) -> (-117.5, -117.5)
  line L461 (-117.5, -117.5) -> (-117.5, 117.5)
  line L462 (-117.5, 117.5) -> (117.5, 117.5)
  line L463 (117.5, 117.5) -> (117.5, -117.5)
  constraint horizontal L460
  constraint vertical L461
  constraint horizontal L462
  constraint vertical L463
  constraint coincident L456.start L459.end
  constraint coincident L457.end L458.start
extrude "Extrude4" [rolled back] along distance 0.2 taper angle 0
extrude "Extrude5" [rolled back] along distance -0.3 taper angle 0
extrude "Extrude6" [rolled back] along distance 8 taper angle 0
sketch "Sketch7" plane through (0, 0, 7) normal (0, 0, 1) x (-1, 0, 0)
  line L0 (42.5, 99.3) -> (57.5, 99.3)
  line L1 (57.5, 99.3) -> (57.5, 114.3)
  line L2 (57.5, 114.3) -> (42.5, 114.3)
  line L3 (42.5, 114.3) -> (42.5, 99.3)
  circle A0 centre (50.0917, 106.8) radius 2.5
  circle A1 centre (16.6917, 106.8) radius 2.5
  circle A2 centre (-16.7083, 106.8) radius 2.5
  circle A3 centre (-50.1083, 106.8) radius 2.5
  dimension "d52" = 5
  dimension "d55" = -33.4
  dimension "d56" = 0
  measures "d52" diameter of A0
extrude "Extrude7" [rolled back] along distance -7 taper angle 0
combine "Combine1" [rolled back]
equation "d12 = 34 mm - ( 16 / 2 ) * 1 mm"
equation "d13 = 35 mm - ( 16 / 2 ) * 1 mm"
equation "d20 = 67.5 mm - ( 15 / 2 ) * 1 mm"
equation "d21 = 10.7 mm - ( 15 / 2 ) * 1 mm"
